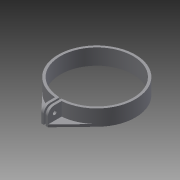
# Autodesk Inventor part: CLAMP
Saved by Autodesk Inventor 2013 (Build 170138000, 138)
## iProperties
Created: 2013-12-22
Part Number: CLAMP
Material: Generic
Document SubType Name: Modeling
Designer: employee
Density: 1 g/cm^3
Mass: 6.0056 g
Surface Area: 69.3101 cm^2
Volume: 6.0056 cm^3
Author: employee
Autodesk Inventor part; units mm, degrees
ref_plane "YZ Plane" through (0, 0, 0) normal (1, 0, 0) x (0, 1, 0)
ref_plane "XZ Plane" through (0, 0, 0) normal (0, 1, 0) x (-1, 0, 0)
ref_plane "XY Plane" through (0, 0, 0) normal (0, 0, 1) x (1, 0, 0)
sketch "Sketch1" plane through (0, 0, 0) normal (0, 0, 1) x (1, 0, 0)
  arc A0 (0.75, -30.1532) -> (-0.75, -30.1532) centre (0, 0) ccw
  arc A1 (2.75, -32.0447) -> (-2.75, -32.0447) centre (0, 0) ccw
  line L0 (-0.75, -30.1532) -> (-0.75, -43.4447)
  line L1 (-0.75, -43.4447) -> (-2.75, -43.4447)
  line L2 (-2.75, -43.4447) -> (-2.75, -32.0447)
  line L3 (0.75, -30.1532) -> (0.75, -43.4447)
  line L4 (0.75, -43.4447) -> (2.75, -43.4447)
  line L5 (2.75, -43.4447) -> (2.75, -32.0447)
  dimension "d0" = 60.325
  dimension "d2" = 2
  dimension "d3" = 2
  dimension "d4" = 1.5
  dimension "d5" = 11.4
  constraints: 12 end point, 4 point on circle, 3 equal length, 3 parallel, 2 centre point, 2 coincident, 2 perpendicular, 1 vertical
  measures "d0" diameter of A0
  measures "d2" radial gap between concentric circles of A1 A0
  measures "d3" distance between parallel lines of L5 L3
  measures "d4" distance between parallel lines of L3 L0
  measures "d5" distance of L4.end L5.end
extrude "Extrusion1" add sketch "Sketch1" along normal blind 11.2
sketch "Sketch2" plane through (2.75, -43.4447, 0) normal (1, 0, 0) x (0, 0, -1)
  line L0 (0, 11.4) -> (-11.2, 11.4) projected
  line L1 (-11.2, 0) -> (-11.2, 11.4) projected
  circle A0 centre (-5.6, 5.7) radius 1.6
  point P0 (0, 43.4447)
  point P1 (-5.6, 11.4)
  point P2 (-11.2, 5.7)
  dimension "d8" = 3.2
  constraints: 2 midpoint, 1 centre point, 1 horizontal alignment, 1 vertical alignment
  measures "d8" diameter of A0
extrude "Extrusion2" cut sketch "Sketch2" against normal through all
sketch "Sketch3" plane through (0, 0, 0) normal (0, 0, -1) x (-1, 0, 0)
  arc A0 (0.75, -30.1532) -> (-0.75, -30.1532) centre (0, 0) ccw projected
  line L0 (0.75, -43.4447) -> (0.75, -30.1532) projected
  line L1 (2.75, -43.4447) -> (0.75, -43.4447) projected
  line L2 (2.75, -32.0447) -> (2.75, -43.4447) projected
  arc A1 (2.75, -32.0447) -> (-2.75, -32.0447) centre (0, 0) ccw projected
  line L3 (-2.75, -43.4447) -> (-2.75, -32.0447) projected
  line L4 (-0.75, -43.4447) -> (-2.75, -43.4447) projected
  line L5 (-0.75, -30.1532) -> (-0.75, -43.4447) projected
extrude "Extrusion3" add sketch "Sketch3" along normal blind 2
sketch "Sketch4" plane through (0, 0, -2) normal (0, 0, -1) x (-1, 0, 0)
  line L0 (2.75, -43.4447) -> (2.75, -32.0447) projected
  arc A0 (2.75, -32.0447) -> (-2.75, -32.0447) centre (0, 0) ccw projected
  line L1 (-2.75, -32.0447) -> (-2.75, -43.4447) projected
  line L2 (2.75, -43.4447) -> (23.1319, -22.346)
  line L3 (-2.75, -43.4447) -> (-23.1319, -22.346)
  constraints: 4 end point, 2 point on circle, 2 tangent
extrude "Extrusion4" add sketch "Sketch4" against normal blind 2
fillet "Fillet1" radius 5.5 2 edges at (1.75, -43.4447, 11.2) (-1.75, -43.4447, 11.2)
fillet "Fillet2" radius 1 4 edges at (-0.75, -30.1532, 5.6) (-0.75, -30.1532, -1) (0.75, -30.1532, 5.6) (0.75, -30.1532, -1)
body "Solid1"
